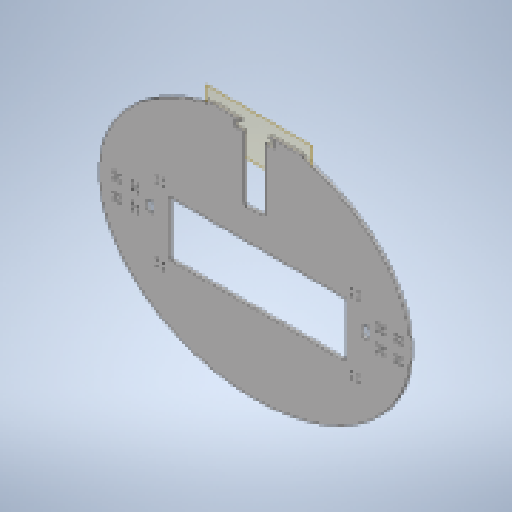
# Autodesk Inventor part: основа_лица
Saved by Autodesk Inventor 2023.1 (Build 271208000, 208)
## iProperties
Created: 2025-02-03
Part Number: основа_лица
Material: Типовые
Document SubType Name: Modeling
Designer: baranovaem
Density: 1 g/cm^3
Appearance: По умолчанию
Author: baranovaem
Autodesk Inventor part; units mm, degrees
ref_plane "YZ Plane" through (0, 0, 0) normal (1, 0, 0) x (0, 1, 0)
ref_plane "XZ Plane" through (0, 0, 0) normal (0, 1, 0) x (-1, 0, 0)
ref_plane "XY Plane" through (0, 0, 0) normal (0, 0, 1) x (1, 0, 0)
ref_plane "РабПлоскость1" through (0, 0, -1.1364) normal (0, 0, 1) x (-1, 0, 0)
sketch "Эскиз2" plane through (0, 0, -1.1364) normal (0, 0, 1) x (-1, 0, 0)
  ellipse E0 centre (4.9908, 190.3029) end of major axis (4.9908, -8.5562) minor radius 260.0344 (84.9908, 1.0887) -> (-75.0092, 1.0887) ccw
  line L0 (84.9908, 1.0887) -> (-75.0092, 1.0887)
  line L1 (-75.0092, 1.0887) -> (-75.0092, -2.9113)
  line L2 (-75.0092, -2.9113) -> (84.9908, -2.9113)
  line L3 (84.9908, -2.9113) -> (84.9908, 1.0887)
  dimension "d206" = 160
  dimension "d207" = 4
  constraints: 8 end point, 2 parallel, 1 horizontal, 1 perpendicular, 4 other
  measures "d206" distance of L2.end L1.end
  measures "d207" distance of L1.end L0.end
extrude "Выдавливание1" add sketch "Эскиз2" along normal mid plane 4
sketch "Эскиз3" plane through (0, 0, -3.1364) normal (0, 0, -1) x (-1, 0, 0)
  line L0 (177.5, -303.2474) -> (-177.5, -303.2474)
  line L1 (-177.5, -303.2474) -> (-177.5, -123.2474)
  line L2 (-177.5, -93.2474) -> (177.5, -93.2474) construction
  line L3 (177.5, -93.2474) -> (177.5, -123.2474) construction
  line L4 (177.5, -303.2474) -> (-177.5, -93.2474) construction
  line L5 (0, 0) -> (0, -505.0871) construction
  line L6 (177.5, -123.2474) -> (-177.5, -123.2474)
  line L7 (177.5, -123.2474) -> (177.5, -303.2474)
  line L8 (-177.5, -123.2474) -> (-177.5, -93.2474) construction
  line L9 (144.5, -258.2474) -> (-144.5, -258.2474)
  line L10 (144.5, -168.2474) -> (-144.5, -168.2474)
  line L11 (147.5, -255.2474) -> (147.5, -171.2474)
  line L12 (-147.5, -255.2474) -> (-147.5, -171.2474)
  arc A0 (144.5, -258.2474) -> (147.5, -255.2474) centre (144.5, -255.2474) ccw
  arc A1 (147.5, -171.2474) -> (144.5, -168.2474) centre (144.5, -171.2474) ccw
  arc A2 (-144.5, -168.2474) -> (-147.5, -171.2474) centre (-144.5, -171.2474) ccw
  arc A3 (-147.5, -255.2474) -> (-144.5, -258.2474) centre (-144.5, -255.2474) ccw
  line L13 (-177.5, -303.2474) -> (177.5, -93.2474) construction
  line L14 (144.5, -255.2474) -> (-144.5, -171.2474) construction
  circle A4 centre (162.5, -153.2474) radius 15 construction
  circle A5 centre (-162.5, -153.2474) radius 15 construction
  circle A6 centre (162.5, -273.2474) radius 15 construction
  circle A7 centre (-162.5, -273.2474) radius 15 construction
  line L15 (144.5, -168.2474) -> (208, -168.2474) construction
  line L16 (147.5, -171.2474) -> (147.5, -106) construction
  line L17 (147.5, -255.2474) -> (147.5, -309) construction
  line L18 (144.5, -258.2474) -> (196, -258.2474) construction
  line L19 (-147.5, -255.2474) -> (-147.5, -298) construction
  line L20 (-144.5, -258.2474) -> (-198, -258.2474) construction
  line L21 (-147.5, -171.2474) -> (-147.5, -131) construction
  line L22 (-144.5, -168.2474) -> (-173, -168.2474) construction
  line L23 (157, -158.2474) -> (168, -158.2474) construction
  line L24 (168, -158.2474) -> (168, -148.2474) construction
  line L25 (168, -148.2474) -> (157, -148.2474) construction
  line L26 (157, -148.2474) -> (157, -158.2474) construction
  line L27 (157, -158.2474) -> (168, -148.2474) construction
  line L28 (168, -158.2474) -> (157, -148.2474) construction
  line L29 (157, -268.2474) -> (168, -268.2474) construction
  line L30 (168, -268.2474) -> (168, -278.2474) construction
  line L31 (168, -278.2474) -> (157, -278.2474) construction
  line L32 (157, -278.2474) -> (157, -268.2474) construction
  line L33 (157, -268.2474) -> (168, -278.2474) construction
  line L34 (168, -268.2474) -> (157, -278.2474) construction
  line L35 (-168, -268.2474) -> (-157, -268.2474) construction
  line L36 (-157, -268.2474) -> (-157, -278.2474) construction
  line L37 (-157, -278.2474) -> (-168, -278.2474) construction
  line L38 (-168, -278.2474) -> (-168, -268.2474) construction
  line L39 (-168, -268.2474) -> (-157, -278.2474) construction
  line L40 (-157, -268.2474) -> (-168, -278.2474) construction
  line L41 (-168, -158.2474) -> (-157, -158.2474) construction
  line L42 (-157, -158.2474) -> (-157, -148.2474) construction
  line L43 (-157, -148.2474) -> (-168, -148.2474) construction
  line L44 (-168, -148.2474) -> (-168, -158.2474) construction
  line L45 (-168, -158.2474) -> (-157, -148.2474) construction
  line L46 (-157, -158.2474) -> (-168, -148.2474) construction
  circle A8 centre (157, -158.2474) radius 1.45
  circle A9 centre (157, -148.2474) radius 1.45
  circle A10 centre (168, -148.2474) radius 1.45
  circle A11 centre (168, -158.2474) radius 1.45
  circle A12 centre (-168, -148.2474) radius 1.45
  circle A13 centre (-157, -148.2474) radius 1.45
  circle A14 centre (-168, -158.2474) radius 1.45
  circle A15 centre (-157, -158.2474) radius 1.45
  circle A16 centre (-157, -268.2474) radius 1.45
  circle A17 centre (-168, -268.2474) radius 1.45
  circle A18 centre (-168, -278.2474) radius 1.45
  circle A19 centre (-157, -278.2474) radius 1.45
  circle A20 centre (168, -278.2474) radius 1.45
  circle A21 centre (168, -268.2474) radius 1.45
  circle A22 centre (157, -268.2474) radius 1.45
  circle A23 centre (157, -278.2474) radius 1.45
  point P0 (0, -198.2474)
  point P1 (-5.6255, -198.2474)
  point P2 (0, -213.2474)
  dimension "d4" = 355
  dimension "d5" = 210
  dimension "d6" = 0
  dimension "d8" = 30
  dimension "d9" = 3
  dimension "d104" = 45
  dimension "d105" = 30
  dimension "d106" = 30
  dimension "d126" = 30
  dimension "d127" = 30
  dimension "d128" = 30
  dimension "d129" = 30
  dimension "d130" = 11
  dimension "d131" = 10
  dimension "d132" = 11
  dimension "d133" = 10
  dimension "d134" = 11
  dimension "d135" = 2.9
  dimension "d136" = 2.9
  dimension "d137" = 2.9
  dimension "d138" = 2.9
  dimension "d139" = 2.9
  dimension "d140" = 2.9
  dimension "d141" = 2.9
  dimension "d142" = 2.9
  dimension "d143" = 2.9
  dimension "d144" = 2.9
  dimension "d145" = 2.9
  dimension "d146" = 2.9
  dimension "d147" = 2.9
  dimension "d148" = 2.9
  dimension "d149" = 2.9
  dimension "d150" = 2.9
  constraints: 94 end point, 24 centre point, 16 coincident, 16 tangent, 14 parallel, 10 midpoint, 10 perpendicular, 9 horizontal, 8 point on circle, 6 vertical, 4 point on line, 3 equal radius
  measures "d4" distance of L0.start L0.end
  measures "d5" distance of L0.end L2.start
  measures "d6" vertical distance of point (-5.625, -198.247) point (0, -198.247)
  measures "d8" distance between parallel lines of L2 L6
  measures "d9" radius of A0
  measures "d104" distance between parallel lines of L0 L9
  measures "d105" distance between parallel lines of L1 L12
  measures "d106" distance between parallel lines of L7 L11
  measures "d126" diameter of A4
  measures "d127" diameter of A5
  measures "d128" diameter of A6
  measures "d129" diameter of A7
  measures "d130" distance of L25.end L24.end
  measures "d131" distance of L24.end L23.end
  measures "d132" distance of L30.end L31.end
  measures "d133" distance of L29.end L30.end
  measures "d134" distance of L36.end L37.end
  measures "d135" diameter of A8
  measures "d136" diameter of A9
  measures "d137" diameter of A10
  measures "d138" diameter of A11
  measures "d139" diameter of A12
  measures "d140" diameter of A13
  measures "d141" diameter of A14
  measures "d142" diameter of A15
  measures "d143" diameter of A16
  measures "d144" diameter of A17
  measures "d145" diameter of A18
  measures "d146" diameter of A19
  measures "d147" diameter of A20
  measures "d148" diameter of A21
  measures "d149" diameter of A22
  measures "d150" diameter of A23
extrude "Выдавливание2" cut sketch "Эскиз3" against normal blind 4 contours L9 A3 L12 A2 L10 A1 L11 A0 | A8 | A9 | A10 | A11 | A12 | A13 | A14 | A15 | A16 | A17 | A18 | A19 | A20 | A21 | A22 | A23
sketch "Эскиз5" plane through (0, 0, -3.1364) normal (0, 0, -1) x (-1, 0, 0)
  ellipse E0 centre (4.9908, -190.3029) end of major axis (265.0252, -190.3029) minor radius 198.8591 (-75.0092, -1.0887) -> (84.9908, -1.0887) ccw projected
  line L0 (84.9908, 2.9113) -> (-75.0092, 2.9113)
  line L1 (-75.0092, 2.9113) -> (-75.0092, -1.0887)
  line L2 (-75.0092, -1.0887) -> (84.9908, -1.0887)
  line L3 (84.9908, -1.0887) -> (84.9908, 2.9113)
  line L4 (-75.0092, 2.9113) -> (84.9908, 2.9113) projected
  line L5 (84.9908, 2.9113) -> (29.9908, 2.9113)
  line L6 (29.9908, 2.9113) -> (29.9908, -1.0887)
  line L7 (29.9908, -1.0887) -> (84.9908, -1.0887)
  line L8 (84.9908, -1.0887) -> (84.9908, 2.9113)
  line L9 (-75.0092, 2.9113) -> (-20.0092, 2.9113)
  line L10 (-20.0092, 2.9113) -> (-20.0092, -1.0887)
  line L11 (-20.0092, -1.0887) -> (-75.0092, -1.0887)
  line L12 (-75.0092, -1.0887) -> (-75.0092, 2.9113)
  point P0 (-20.0092, 2.9113)
  point P1 (29.9908, 2.9113)
  dimension "d208" = 55
  dimension "d209" = 55
  constraints: 24 end point, 6 parallel, 3 horizontal, 3 perpendicular, 2 point on line, 2 other
  measures "d208" distance of L7.end L6.end
  measures "d209" distance of L10.end L11.end
extrude "Выдавливание4" cut sketch "Эскиз5" against normal blind 4 contours L10 L0 L6 L2
sketch "Эскиз6" plane through (0, 0, 0.8636) normal (0, 0, 1) x (1, 0, 0)
  line L0 (-84.9908, -1.0887) -> (-84.9908, 2.9113) projected
  line L1 (75.0092, -1.0887) -> (-84.9908, -1.0887) construction
  line L2 (-4.9908, -1.0887) -> (-4.9908, -151.6518) construction
  line L3 (10.0092, -117.0887) -> (-19.9908, -117.0887)
  line L4 (-21.9908, -115.0887) -> (-21.9908, 2.9113)
  line L5 (-21.9908, 2.9113) -> (12.0092, 2.9113)
  line L6 (12.0092, 2.9113) -> (12.0092, -115.0887)
  line L7 (12.0092, -117.0887) -> (-21.9908, 2.9113) construction
  line L8 (-21.9908, -117.0887) -> (12.0092, 2.9113) construction
  line L9 (20.0092, 2.9113) -> (75.0092, 2.9113) construction
  line L10 (-84.9908, 2.9113) -> (-29.9908, 2.9113) construction
  line L11 (20.0092, 2.9113) -> (-29.9908, 2.9113) construction
  arc A0 (10.0092, -117.0887) -> (12.0092, -115.0887) centre (10.0092, -115.0887) ccw
  arc A1 (-21.9908, -115.0887) -> (-19.9908, -117.0887) centre (-19.9908, -115.0887) ccw
  line L12 (12.0092, -1.0887) -> (27.0092, -1.0887)
  line L13 (27.0092, -1.0887) -> (27.0092, -11.0887)
  line L14 (27.0092, -11.0887) -> (12.0092, -11.0887)
  line L15 (12.0092, -11.0887) -> (12.0092, -1.0887)
  line L16 (-21.9908, -1.0887) -> (-36.9908, -1.0887)
  line L17 (-36.9908, -1.0887) -> (-36.9908, -11.0887)
  line L18 (-36.9908, -11.0887) -> (-21.9908, -11.0887)
  line L19 (-21.9908, -11.0887) -> (-21.9908, -1.0887)
  point P0 (-4.9908, -57.0887)
  point P1 (-4.9908, 2.9113)
  point P2 (-21.9908, -11.0887)
  point P3 (12.0092, -11.0887)
  point P4 (20.0092, -1.0887)
  point P5 (-29.4908, -1.0887)
  dimension "d210" = 34
  dimension "d211" = 120
  dimension "d212" = 2
  dimension "d213" = 15
  dimension "d214" = 10
  dimension "d215" = 15
  dimension "d216" = 10
  constraints: 34 end point, 8 point on line, 6 parallel, 5 horizontal, 5 midpoint, 4 point on circle, 4 tangent, 3 perpendicular, 2 centre point, 1 equal radius, 1 vertical
  measures "d210" distance of L4.end L5.end
  measures "d211" distance of L8.start L4.end
  measures "d212" radius of A0
  measures "d213" distance of L13.end L14.end
  measures "d214" distance of L12.end L13.end
  measures "d215" distance of L18.end L17.end
  measures "d216" distance of L17.end L16.end
extrude "Выдавливание5" cut sketch "Эскиз6" against normal blind 4
sketch "Эскиз9" plane through (0, 0, -3.1364) normal (0, 0, -1) x (-1, 0, 0)
  line L0 (-235, -202.49) -> (-235, -223.51) construction
  circle A0 centre (217.2499, 89.3506) radius 1.6806
  circle A1 centre (212.1896, 94.5548) radius 3.0463
  circle A2 centre (217.3783, 99.3507) radius 1.6805
  circle A3 centre (206.8799, 99.3342) radius 1.6809
  circle A4 centre (206.8954, 89.3342) radius 1.6807
  circle A5 centre (217.2499, 89.3506) radius 1.6806
  circle A6 centre (212.1896, 94.5548) radius 3.0463
  circle A7 centre (217.3783, 99.3507) radius 1.6805
  circle A8 centre (206.8799, 99.3342) radius 1.6809
  circle A9 centre (206.8954, 89.3342) radius 1.6807
  circle A10 centre (-235, -213) radius 3
  line L1 (-230, -218.25) -> (-240, -218.25) construction
  line L2 (-240, -218.25) -> (-240, -207.75) construction
  line L3 (-240, -207.75) -> (-230, -207.75) construction
  line L4 (-230, -207.75) -> (-230, -218.25) construction
  line L5 (-230, -218.25) -> (-240, -207.75) construction
  line L6 (-240, -218.25) -> (-230, -207.75) construction
  circle A11 centre (-240, -218.25) radius 1.65
  circle A12 centre (-240, -207.75) radius 1.65
  circle A13 centre (-230, -207.75) radius 1.65
  circle A14 centre (-230, -218.25) radius 1.65
  circle A15 centre (-205, -213) radius 3
  line L7 (-200, -218.25) -> (-210, -218.25) construction
  line L8 (-210, -218.25) -> (-210, -207.75) construction
  line L9 (-210, -207.75) -> (-200, -207.75) construction
  line L10 (-200, -207.75) -> (-200, -218.25) construction
  line L11 (-200, -218.25) -> (-210, -207.75) construction
  line L12 (-210, -218.25) -> (-200, -207.75) construction
  circle A16 centre (-210, -218.25) radius 1.65
  circle A17 centre (-210, -207.75) radius 1.65
  circle A18 centre (-200, -207.75) radius 1.65
  circle A19 centre (-200, -218.25) radius 1.65
  circle A20 centre (-235, -183) radius 3
  line L13 (-230, -188.25) -> (-240, -188.25) construction
  line L14 (-240, -188.25) -> (-240, -177.75) construction
  line L15 (-240, -177.75) -> (-230, -177.75) construction
  line L16 (-230, -177.75) -> (-230, -188.25) construction
  line L17 (-230, -188.25) -> (-240, -177.75) construction
  line L18 (-240, -188.25) -> (-230, -177.75) construction
  circle A21 centre (-240, -188.25) radius 1.65
  circle A22 centre (-240, -177.75) radius 1.65
  circle A23 centre (-230, -177.75) radius 1.65
  circle A24 centre (-230, -188.25) radius 1.65
  line L19 (-147.5, -255.2474) -> (-147.5, -171.2474) projected
  line L20 (0, 0) -> (0, -408.2262) construction
  line L21 (-200, -177.75) -> (-200, -188.25) construction
  circle A25 centre (-205, -183) radius 3
  line L22 (-210, -177.75) -> (-200, -177.75) construction
  line L23 (-200, -188.25) -> (-210, -177.75) construction
  line L24 (-210, -188.25) -> (-200, -177.75) construction
  line L25 (-200, -188.25) -> (-210, -188.25) construction
  line L26 (-210, -188.25) -> (-210, -177.75) construction
  circle A26 centre (-210, -188.25) radius 1.65
  circle A27 centre (-210, -177.75) radius 1.65
  circle A28 centre (-200, -177.75) radius 1.65
  circle A29 centre (-200, -188.25) radius 1.65
  line L27 (235, -202.49) -> (235, -223.51) construction
  circle A30 centre (235, -213) radius 3
  line L28 (230, -218.25) -> (240, -218.25) construction
  line L29 (240, -218.25) -> (240, -207.75) construction
  line L30 (240, -207.75) -> (230, -207.75) construction
  line L31 (230, -207.75) -> (230, -218.25) construction
  line L32 (230, -218.25) -> (240, -207.75) construction
  line L33 (240, -218.25) -> (230, -207.75) construction
  circle A31 centre (240, -218.25) radius 1.65
  circle A32 centre (240, -207.75) radius 1.65
  circle A33 centre (230, -207.75) radius 1.65
  circle A34 centre (230, -218.25) radius 1.65
  line L34 (200, -207.75) -> (200, -218.25) construction
  circle A35 centre (205, -213) radius 3
  line L35 (210, -207.75) -> (200, -207.75) construction
  line L36 (200, -218.25) -> (210, -207.75) construction
  line L37 (210, -218.25) -> (200, -207.75) construction
  line L38 (200, -218.25) -> (210, -218.25) construction
  line L39 (210, -218.25) -> (210, -207.75) construction
  circle A36 centre (210, -218.25) radius 1.65
  circle A37 centre (210, -207.75) radius 1.65
  circle A38 centre (200, -207.75) radius 1.65
  circle A39 centre (200, -218.25) radius 1.65
  line L40 (230, -177.75) -> (230, -188.25) construction
  circle A40 centre (235, -183) radius 3
  line L41 (240, -177.75) -> (230, -177.75) construction
  line L42 (230, -188.25) -> (240, -177.75) construction
  line L43 (240, -188.25) -> (230, -177.75) construction
  line L44 (230, -188.25) -> (240, -188.25) construction
  line L45 (240, -188.25) -> (240, -177.75) construction
  circle A41 centre (240, -188.25) radius 1.65
  circle A42 centre (240, -177.75) radius 1.65
  circle A43 centre (230, -177.75) radius 1.65
  circle A44 centre (230, -188.25) radius 1.65
  line L46 (200, -188.25) -> (210, -188.25) construction
  circle A45 centre (210, -188.25) radius 1.65
  line L47 (210, -188.25) -> (210, -177.75) construction
  circle A46 centre (210, -177.75) radius 1.65
  line L48 (200, -177.75) -> (200, -188.25) construction
  line L49 (200, -188.25) -> (210, -177.75) construction
  line L50 (210, -188.25) -> (200, -177.75) construction
  line L51 (210, -177.75) -> (200, -177.75) construction
  circle A47 centre (200, -177.75) radius 1.65
  circle A48 centre (200, -188.25) radius 1.65
  circle A49 centre (205, -183) radius 3
  ellipse E0 centre (180, -198) end of major axis (180, -188) minor radius 6
  ellipse E1 centre (-180, -200) end of major axis (-180, -190) minor radius 6
  dimension "d152" = 6
  dimension "d153" = 10
  dimension "d155" = 6
  dimension "d156" = 10
  dimension "d52" = 6
  dimension "d53" = 10
  dimension "d54" = 10.5
  dimension "d55" = 3.3
  dimension "d56" = 3.3
  dimension "d57" = 3.3
  dimension "d58" = 6
  dimension "d59" = 10
  dimension "d60" = 10.5
  dimension "d61" = 3.3
  dimension "d62" = 3.3
  dimension "d63" = 3.3
  dimension "d64" = 6
  dimension "d65" = 10
  dimension "d66" = 10.5
  dimension "d67" = 3.3
  dimension "d68" = 3.3
  dimension "d69" = 3.3
  dimension "d70" = 30
  dimension "d71" = 30
  dimension "d97" = 235
  dimension "d98" = 6
  dimension "d99" = 10
  dimension "d100" = 10.5
  dimension "d101" = 3.3
  dimension "d102" = 3.3
  dimension "d103" = 3.3
  dimension "d154" = 20
  dimension "d157" = 20
  constraints: 102 end point, 50 centre point, 38 symmetric about line, 32 coincident, 9 midpoint, 8 parallel, 4 horizontal, 4 perpendicular, 1 vertical, 24 other
  measures "d52" diameter of A10
  measures "d53" distance of L2.end L3.end
  measures "d54" distance of L3.end L1.start
  measures "d55" diameter of A11
  measures "d56" diameter of A12
  measures "d57" diameter of A14
  measures "d58" diameter of A15
  measures "d59" distance of L9.start L10.start
  measures "d60" distance of L10.start L10.end
  measures "d61" diameter of A16
  measures "d62" diameter of A17
  measures "d63" diameter of A19
  measures "d64" diameter of A20
  measures "d65" distance of L15.start L16.start
  measures "d66" distance of L16.start L16.end
  measures "d67" diameter of A21
  measures "d68" diameter of A22
  measures "d69" diameter of A24
  measures "d70" distance of A15.centre A10.centre
  measures "d71" distance of A20.centre A10.centre
  measures "d97" distance from line of L20 A10.centre
  measures "d98" diameter of A25
  measures "d99" distance of L26.end L21.start
  measures "d100" distance of L21.start L25.start
  measures "d101" diameter of A26
  measures "d102" diameter of A27
  measures "d103" diameter of A29
  measures "d154" horizontal distance of point (180, -198) L34.start
  measures "d157" horizontal distance of L10.start point (-180, -200)
extrude "Выдавливание8" cut sketch "Эскиз9" against normal blind 4 contours A10 | A11 | A12 | A13 | A14 | A15 | A16 | A17 | A18 | A19 | A20 | A21 | A22 | A23 | A24 | A25 | A26 | A27 | A28 | A29 | A30 | A31 | A32 | A33 | A34 | A35 | A36 | A37 | A38 | A39 | A40 | A41 | A42 | A43 | A44 | A45 | A46 | A47 | A48 | A49 | E0 | E1
